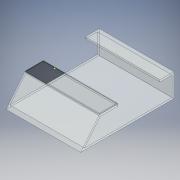
# Autodesk Inventor part: Bottom Plastic
Saved by Autodesk Inventor 2018 (Build 220112000, 112)
## iProperties
Created: 2018-02-19
Part Number: Bottom Plastic
Material: Generic
Document SubType Name: Modeling
Designer: Melda
Density: 1 g/cm^3
Appearance: Clear
Author: Melda
Autodesk Inventor part; units mm, degrees
ref_plane "YZ Plane" through (0, 0, 0) normal (1, 0, 0) x (0, 1, 0)
ref_plane "XZ Plane" through (0, 0, 0) normal (0, 1, 0) x (-1, 0, 0)
ref_plane "XY Plane" through (0, 0, 0) normal (0, 0, 1) x (1, 0, 0)
sketch "Sketch1" plane through (0, 0, 0) normal (1, 0, 0) x (0, 1, 0)
  point P0 (0, 0)
sketch "Sketch2" plane through (0, 0, 0) normal (1, 0, 0) x (0, 1, 0)
  line L0 (25.8289, -95.4545) -> (-24.1711, -95.4545)
  line L1 (-24.1711, -95.4545) -> (-24.1711, 104.5455)
  line L2 (-24.1711, 104.5455) -> (25.8289, 64.5455)
  line L3 (25.8289, 64.5455) -> (25.8289, 24.5455)
  line L4 (25.8289, -95.4545) -> (25.8289, -65.4545)
  line L5 (21.8289, -91.4545) -> (-20.1711, -91.4545)
  line L6 (-20.1711, -91.4545) -> (-20.1711, 24.5455)
  line L7 (21.8289, 62.623) -> (-20.1711, 96.223)
  line L8 (-20.1711, 96.223) -> (-20.1711, 24.5455)
  line L9 (25.8289, 24.5455) -> (21.8289, 24.5455)
  line L10 (25.8289, -65.4545) -> (21.8289, -65.4545)
  line L11 (21.8289, 62.623) -> (21.8289, 24.5455)
  line L12 (21.8289, -65.4545) -> (21.8289, -91.4545)
  point P0 (0, 0)
  dimension "d3" = 200
  dimension "d4" = 40
  dimension "d5" = 50
  dimension "d6" = 30
  dimension "d7" = 40
  dimension "d9" = 51.34
  dimension "d10" = 4
  dimension "d12" = 4
  dimension "d14" = 4
  dimension "d15" = 4
  dimension "d16" = 4
  dimension "d17" = 4
  dimension "d18" = 4
  constraints: 26 end point, 5 perpendicular, 4 parallel, 2 vertical, 1 horizontal, 1 point on line
  measures "d3" distance of L0.end L1.end
  measures "d4" vertical distance of L1.end L2.end
  measures "d5" distance of L0.start L0.end
  measures "d6" distance of L0.start L4.end
  measures "d7" distance of L2.end L3.end
  measures "d9" angle of L1 L2
  measures "d10" distance of L4.end L10.end
  measures "d12" distance between parallel lines of L1 L6
  measures "d14" distance from line of L2 L7.end
  measures "d15" distance of L3.end L9.end
  measures "d16" distance from line of L2 L7.start
  measures "d17" distance from line of L0 L5.start
  measures "d18" distance from line of L0 L5.end
extrude "Extrusion1" add sketch "Sketch2" along normal blind 160
sketch "Sketch3" plane through (0, 25.8289, 64.5455) normal (0, 1, 0) x (1, 0, 0)
  line L0 (1, 1) -> (159, 1)
  line L1 (159, 1) -> (159, 39)
  line L2 (159, 39) -> (1, 39)
  line L3 (1, 39) -> (1, 1)
  line L4 (0, 40) -> (0, 0) projected
  line L5 (0, 40) -> (160, 40) projected
  line L6 (0, 0) -> (160, 0) projected
  line L7 (160, 40) -> (160, 0) projected
  point P0 (0, 64.5455)
  dimension "d21" = 1
  dimension "d22" = 1
  dimension "d23" = 1
  dimension "d24" = 1
  constraints: 8 end point, 6 parallel, 1 horizontal, 1 perpendicular
  measures "d21" distance between parallel lines of L4 L3
  measures "d22" distance between parallel lines of L5 L2
  measures "d23" distance between parallel lines of L6 L0
  measures "d24" distance between parallel lines of L7 L1
extrude "Extrusion2" add sketch "Sketch3" along normal blind 2 contours L3 L2 L1 L0
sketch "Sketch5" plane through (0, 0, 0) normal (-1, 0, 0) x (0, 0, 1)
  point P0 (0, 0)
body "Solid1"
